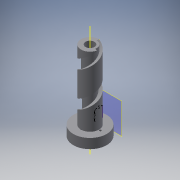
# Autodesk Inventor part: ScrewActuatorGripper
Saved by Autodesk Inventor 2018 (Build 220112000, 112)
## iProperties
Created: 2016-10-16
Part Number: ScrewActuatorGripper
Material: Generic
Document SubType Name: Modeling
Designer: Bardo91
Density: 1 g/cm^3
Appearance: Default
Author: Bardo91
Autodesk Inventor part; units mm, degrees
ref_plane "YZ Plane" through (0, 0, 0) normal (1, 0, 0) x (0, 1, 0)
ref_plane "XY Plane" through (0, 0, 0) normal (0, 0, 1) x (1, 0, 0)
sketch "Sketch1" plane through (0, 0, 0) normal (0, 0, 1) x (1, 0, 0)
  line L0 (0, 0) -> (0, 7.5)
  circle A0 centre (0, 7.5) radius 1.5
  circle A1 centre (-5.3033, 5.3033) radius 1.5
  circle A2 centre (-7.5, 0) radius 1.5
  circle A3 centre (-5.3033, -5.3033) radius 1.5
  circle A4 centre (0, -7.5) radius 1.5
  circle A5 centre (5.3033, -5.3033) radius 1.5
  circle A6 centre (7.5, 0) radius 1.5
  circle A7 centre (5.3033, 5.3033) radius 1.5
  circle A8 centre (0, 0) radius 12
  dimension "d0" = 7.5
  dimension "d1" = 3
  dimension "d4" = 360
  dimension "d6" = 24
  constraints: 9 centre point, 2 coincident, 2 end point, 1 vertical, 17 other
  measures "d0" distance of L0.start L0.end
  measures "d1" diameter of A0
  measures "d6" diameter of A8
extrude "Extrusion1" add sketch "Sketch1" along normal blind 7 contours A1 | A3 | A5 | A7 | A8
sketch "Sketch2" plane through (0, 0, 0) normal (0, 0, -1) x (-1, 0, 0)
  circle A0 centre (0, 0) radius 6.5
  dimension "d9" = 13
  constraints: 1 centre point, 1 coincident
  measures "d9" diameter of A0
extrude "Extrusion2" cut sketch "Sketch2" against normal blind 1
sketch "Sketch3" plane through (0, 0, 7) normal (0, 0, 1) x (1, 0, 0)
  circle A0 centre (0, 0) radius 6.5
  dimension "d12" = 13
  constraints: 1 centre point, 1 coincident
  measures "d12" diameter of A0
extrude "Extrusion3" add sketch "Sketch3" along normal blind 50
sketch "Sketch5" plane through (0, 0, 57) normal (0, 0, 1) x (1, 0, 0)
  circle A0 centre (0, 0) radius 3.25
  dimension "d25" = 6.5
  constraints: 1 centre point, 1 coincident
  measures "d25" diameter of A0
extrude "Extrusion5" cut sketch "Sketch5" against normal up to surface (56 mm away)
ref_plane "Work Plane1" through (0, 12, 0) normal (0, 1, 0) x (-1, 0, 0)
sketch "Sketch8" plane through (0, 0, 7) normal (0, 0, 1) x (1, 0, 0)
  circle A0 centre (0, 0) radius 3
  dimension "d44" = 6
  constraints: 1 centre point, 1 coincident
  measures "d44" diameter of A0
extrude "Extrusion8" cut sketch "Sketch8" against normal through all
sketch "Sketch9" plane through (0, 0, 0) normal (1, 0, 0) x (0, 1, 0)
  line L0 (6.5, 7) -> (6.5, 57) projected
  line L1 (6.5, 7) -> (6.5, 57) projected
  line L2 (6.4167, 7) -> (9, 7) projected
  line L3 (9, 7) -> (4, 7)
  line L4 (4, 7) -> (4, 14)
  line L5 (4, 14) -> (9, 14)
  line L6 (9, 14) -> (9, 7)
  line L7 (0, -11.4) -> (0, 68.4) projected
  point P0 (0, 0)
  dimension "d61" = 5
  dimension "d62" = 7
  constraints: 8 end point, 2 parallel, 1 horizontal, 1 perpendicular
  measures "d61" distance of L4.end L5.end
  measures "d62" distance of L3.end L4.end
coil "Coil2" sketch "Sketch9" operation cut axis through (0, 0, 7) along (0, 0, 1) pitch 25 turns 2 hand right taper 1
sketch "Boceto13" plane through (0, 0, 0) normal (0, 0, -1) x (-1, 0, 0)
  arc A0 (-6.4167, 1.0375) -> (-6.4167, -1.0375) centre (-7.5, 0) ccw projected
  circle A1 centre (-7.5, 0) radius 1.5
  arc A2 (-1.0375, -6.4167) -> (1.0375, -6.4167) centre (0, -7.5) ccw projected
  circle A3 centre (0, -7.5) radius 1.5
  arc A4 (1.0375, 6.4167) -> (-1.0375, 6.4167) centre (0, 7.5) ccw projected
  circle A5 centre (0, 7.5) radius 1.5
  arc A6 (6.4167, -1.0375) -> (6.4167, 1.0375) centre (7.5, 0) ccw projected
  circle A7 centre (7.5, 0) radius 1.5
  point P0 (0, 0)
  constraints: 4 centre point, 4 coincident
extrude "Extrusión9" add sketch "Boceto13" against normal blind 7
sketch "Boceto14" plane through (0, 0, 1) normal (0, 0, -1) x (-1, 0, 0)
  circle A0 centre (0, 0) radius 6.5
  constraints: 1 centre point, 1 coincident
extrude "Extrusión10" cut sketch "Boceto14" along normal blind 2
sketch "Boceto15" plane through (0, 0, 0) normal (0, 0, -1) x (-1, 0, 0)
  line L0 (0, 0) -> (-7.5, 0)
  line L1 (0, 0) -> (7.5, 0)
  line L2 (0, 0) -> (0, 6)
  line L3 (0, 0) -> (0, -6)
  circle A0 centre (0, 6) radius 0.75
  circle A1 centre (-7.5, 0) radius 0.75
  circle A2 centre (0, -6) radius 0.75
  circle A3 centre (7.5, 0) radius 0.75
  dimension "d76" = 7.5
  dimension "d77" = 7.5
  dimension "d78" = 6
  dimension "d79" = 6
  dimension "d80" = 1.5
  dimension "d81" = 1.5
  dimension "d82" = 1.5
  dimension "d83" = 1.5
  constraints: 8 end point, 4 centre point, 4 coincident, 2 horizontal, 2 vertical
  measures "d76" distance of L0.start L0.end
  measures "d77" distance of L0.start L1.end
  measures "d78" distance of L0.start L2.end
  measures "d79" distance of L0.start L3.end
  measures "d80" diameter of A0
  measures "d81" diameter of A1
  measures "d82" diameter of A2
  measures "d83" diameter of A3
extrude "Extrusión11" cut sketch "Boceto15" against normal blind 7
body "Solid1"
